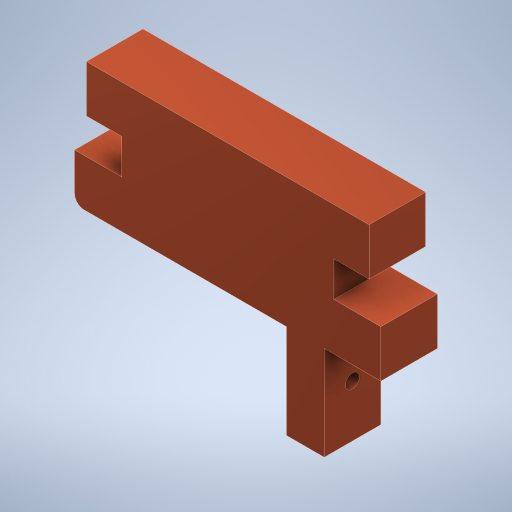
# Autodesk Inventor part: Basegripper
Saved by Autodesk Inventor 2024 (Build 280153000, 153)
## iProperties
Created: 2023-12-04
Part Number: Basegripper
Material: Copper, Wrought
Document SubType Name: Modeling
Designer: Juan_Daleman
Density: 8.94 g/cm^3
Appearance: Copper - Satin
Author: Juan_Daleman
Autodesk Inventor part; units mm, degrees
ref_plane "YZ Plane" through (0, 0, 0) normal (1, 0, 0) x (0, 1, 0)
ref_plane "XZ Plane" through (0, 0, 0) normal (0, 1, 0) x (-1, 0, 0)
ref_plane "XY Plane" through (0, 0, 0) normal (0, 0, 1) x (1, 0, 0)
sketch "Sketch1" plane through (0, 0, 0) normal (0, 0, 1) x (1, 0, 0)
  line L0 (0, 0) -> (0, 10)
  line L1 (0, 10) -> (60, 10)
  line L2 (60, 10) -> (60, 0)
  line L3 (0, 0) -> (7.5, 0)
  line L4 (7.5, 0) -> (7.5, -7.5)
  line L5 (7.5, -7.5) -> (-2.5, -7.5)
  line L6 (-2.5, -7.5) -> (-2.5, -17.5)
  line L7 (30, 10) -> (30, -7.5) construction
  line L8 (60, 0) -> (52.5, 0)
  line L9 (52.5, 0) -> (52.5, -7.5)
  line L10 (52.5, -7.5) -> (62.5, -7.5)
  line L11 (62.5, -7.5) -> (62.5, -17.5)
  line L12 (62.5, -17.5) -> (50.5, -17.5)
  line L13 (50.5, -17.5) -> (50.5, -37.5)
  line L14 (50.5, -37.5) -> (42.5, -37.5)
  line L15 (42.5, -37.5) -> (42.5, -17.5)
  line L16 (42.5, -17.5) -> (-2.5, -17.5)
  dimension "d0" = 10
  dimension "d2" = 60
  dimension "d3" = 7.5
  dimension "d4" = 7.5
  dimension "d5" = 10
  dimension "d6" = 10
  dimension "d21" = 12
  dimension "d22" = 20
  dimension "d23" = 8
  constraints: 34 end point, 7 perpendicular, 4 symmetric about line, 3 horizontal, 3 vertical, 1 midpoint, 1 point on line
  measures "d0" distance of L0.start L0.end
  measures "d2" distance of L0.end L1.end
  measures "d3" distance of L0.start L3.end
  measures "d4" distance of L3.end L4.end
  measures "d5" distance of L4.end L5.end
  measures "d6" distance of L5.end L6.end
  measures "d21" distance of L11.end L12.end
  measures "d22" distance of L12.end L13.end
  measures "d23" distance of L13.end L14.end
extrude "Extrusion1" add sketch "Sketch1" along normal blind 12
sketch "Sketch2" plane through (50.5, -37.5, 0) normal (1, 0, 0) x (0, 0, -1)
  line L0 (0, 20) -> (0, 30) projected
  line L1 (0, 0) -> (0, 20) projected
  line L2 (-12, 0) -> (-12, 8) projected
  line L3 (0, 0) -> (-12, 0) projected
  line L4 (0, 0) -> (-6, 0)
  line L5 (-6, 0) -> (-6, 20)
  line L6 (-6, 20) -> (-6, 17)
  line L7 (-6, 17) -> (-6, 11)
  circle A0 centre (-6, 17) radius 1.5
  circle A1 centre (-6, 11) radius 1.5
  point P0 (0, 37.5)
  dimension "d24" = 6
  dimension "d27" = 3
  dimension "d28" = 6
  dimension "d29" = 3
  dimension "d30" = 3
  constraints: 8 end point, 2 centre point, 2 coincident, 2 point on line, 1 midpoint, 1 vertical
  measures "d24" distance of L1.start L4.end
  measures "d27" distance of L5.end L6.end
  measures "d28" distance of L6.end L7.end
  measures "d29" diameter of A0
  measures "d30" diameter of A1
extrude "Extrusion2" cut sketch "Sketch2" against normal through all
fillet "Fillet1" radius 2 1 edges at (-2.5, -17.5, 6)
body "Solid1"
